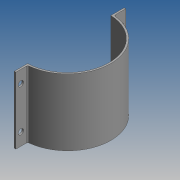
# Autodesk Inventor part: P050_SupportTube2
Saved by Autodesk Inventor 2021.3 (Build 253353000, 353)
## iProperties
Created: 2022-01-14
Part Number: P050_SupportTube2
Material: Générique
Document SubType Name: Modeling
Designer: gabri
Density: 1 g/cm^3
Appearance: Par défaut
Author: gabri
Autodesk Inventor part; units mm, degrees
ref_plane "YZ Plane" through (0, 0, 0) normal (1, 0, 0) x (0, 1, 0)
ref_plane "XZ Plane" through (0, 0, 0) normal (0, 1, 0) x (-1, 0, 0)
ref_plane "XY Plane" through (0, 0, 0) normal (0, 0, 1) x (1, 0, 0)
sketch "Sketch2" plane through (0, 0, 0) normal (0, 0, 1) x (1, 0, 0)
  arc A0 (0, -52) -> (0, 52) centre (0, 0) ccw
  arc A1 (0, -50) -> (0, 50) centre (0, 0) ccw
  line L0 (0, 52) -> (0, 50)
  line L1 (0, -50) -> (0, -52)
  line L2 (2, 49.96) -> (4, 49.96)
  line L3 (4, 49.96) -> (4, 65.96)
  line L4 (4, 65.96) -> (2, 65.96)
  line L5 (2, 65.96) -> (2, 49.96)
  line L6 (2, -49.96) -> (4, -49.96)
  line L7 (4, -49.96) -> (4, -65.96)
  line L8 (4, -65.96) -> (2, -65.96)
  line L9 (2, -65.96) -> (2, -49.96)
  line L10 (0, 92.344) -> (0, -92.344) construction
  point P0 (4, -51.8459)
  point P1 (4, 51.8459)
  dimension "d0" = 104
  dimension "d1" = 100
  dimension "d2" = 2
  dimension "d40" = 2
  dimension "d41" = 2
  dimension "d42" = 16
  dimension "d43" = 16
  dimension "d44" = 2
  dimension "d45" = 2
  constraints: 20 end point, 6 point on circle, 4 parallel, 2 centre point, 2 coincident, 2 horizontal, 2 perpendicular, 2 point on line, 1 vertical
  measures "d0" diameter of A0
  measures "d1" diameter of A1
  measures "d2" distance of L0.start L0.end
  measures "d40" distance between parallel lines of L10 L9
  measures "d41" distance between parallel lines of L9 L7
  measures "d42" distance between parallel lines of L6 L8
  measures "d43" distance between parallel lines of L2 L4
  measures "d44" distance between parallel lines of L10 L5
  measures "d45" distance between parallel lines of L5 L3
extrude "Extrusion1" add sketch "Sketch2" along normal blind 80 contours L9 L6 L7 A0 | A0 L7 L8 L9 | L7 L6 A1 L2 L3 A0 | L3 L2 L5 A0 | A0 L5 L4 L3
fillet "Fillet4" radius 2 2 edges at (4, 51.8459, 40) (4, -51.8459, 40)
sketch "Sketch6" plane through (4, -65.96, 80) normal (1, 0, 0) x (0, 0, -1)
  line L0 (80, 16) -> (80, 0) construction
  line L1 (80, 0) -> (0, 0) construction
  line L2 (0, 16) -> (0, 0) construction
  line L3 (80, 16) -> (0, 16) construction
  line L4 (80, 131.92) -> (80, 115.92) construction
  line L5 (80, 115.92) -> (0, 115.92) construction
  line L6 (0, 131.92) -> (0, 115.92) construction
  line L7 (80, 131.92) -> (0, 131.92) construction
  point P0 (80, 65.96)
  point P1 (15, 6)
  point P2 (65, 6)
  point P3 (65, 125.92)
  point P4 (15, 125.92)
  dimension "d47" = 15
  dimension "d48" = 15
  dimension "d49" = 15
  dimension "d50" = 15
  dimension "d51" = 6
  dimension "d52" = 6
  dimension "d53" = 6
  dimension "d54" = 6
  measures "d47" distance from line of L2 point (15, 6)
  measures "d48" distance from line of L0 point (65, 6)
  measures "d49" distance from line of L4 point (65, 125.92)
  measures "d50" distance from line of L6 point (15, 125.92)
  measures "d51" distance from line of L1 point (15, 6)
  measures "d52" distance from line of L1 point (65, 6)
  measures "d53" distance from line of L7 point (65, 125.92)
  measures "d54" distance from line of L7 point (15, 125.92)
hole "Hole3" at (4, -59.96, 65) at (4, -59.96, 15) at (4, 59.96, 15) at (4, 59.96, 65) direction (-1, 0, 0) diameter 6.5 depth 2
body "Solid1"
